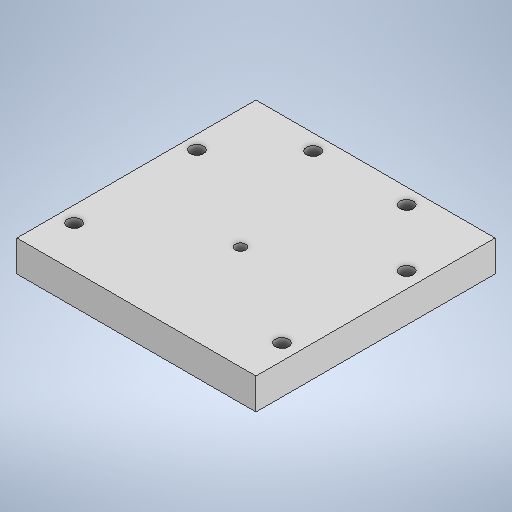
# Autodesk Inventor part: Part_side
Saved by Autodesk Inventor 2025 (Build 290162010, 162A)
## iProperties
Created: 2024-07-05
Part Number: Part_side
Material: Generic
Document SubType Name: Modeling
Designer: kani2
Density: 1 g/cm^3
Appearance: Default
Author: kani2
Autodesk Inventor part; units mm, degrees
ref_plane "YZ Plane" through (0, 0, 0) normal (1, 0, 0) x (0, 1, 0)
ref_plane "XZ Plane" through (0, 0, 0) normal (0, 1, 0) x (-1, 0, 0)
ref_plane "XY Plane" through (0, 0, 0) normal (0, 0, 1) x (1, 0, 0)
sketch "Sketch1" plane through (0, 0, 0) normal (0, 1, 0) x (-1, 0, 0)
  line L0 (73.025, 73.025) -> (-73.025, 73.025)
  line L1 (-73.025, 73.025) -> (-73.025, -73.025)
  line L2 (-73.025, -73.025) -> (73.025, -73.025)
  line L3 (73.025, -73.025) -> (73.025, 73.025)
  line L4 (73.025, 73.025) -> (-73.025, -73.025) construction
  line L5 (-73.025, 73.025) -> (73.025, -73.025) construction
  point P0 (0, 0)
  dimension "d2" = 146.05
  dimension "d3" = 146.05
  constraints: 12 end point, 2 midpoint, 2 parallel, 1 horizontal, 1 perpendicular
  measures "d2" distance of L2.end L1.end
  measures "d3" distance of L1.end L0.end
extrude "Extrusion1" add sketch "Sketch1" along normal blind 19.05
sketch "Sketch2" plane through (0, 19.05, 0) normal (0, 1, 0) x (1, 0, 0)
  circle A0 centre (0, -9.525) radius 3.175
  line L0 (73.025, 73.025) -> (-73.025, 73.025) projected
  line L1 (-73.025, 73.025) -> (-73.025, -73.025) projected
  point P0 (0, 0)
  dimension "d6" = 6.35
  dimension "d7" = 82.55
  dimension "d8" = 73.025
  constraints: 1 centre point
  measures "d6" diameter of A0
  measures "d7" distance from line of L0 A0.centre
  measures "d8" distance from line of L1 A0.centre
extrude "Extrusion2" cut sketch "Sketch2" against normal blind 19.05
sketch "Sketch3" plane through (0, 19.05, 0) normal (0, 1, 0) x (1, 0, 0)
  circle A0 centre (-63.5, -47.625) radius 4.0894
  line L0 (-73.025, 73.025) -> (-73.025, -73.025) projected
  line L1 (-73.025, -73.025) -> (73.025, -73.025) projected
  circle A1 centre (-64.6763, 28.575) radius 4.0894
  circle A2 centre (63.5, -47.625) radius 4.0894
  line L2 (73.025, -73.025) -> (73.025, 73.025) projected
  circle A3 centre (63.5, 28.575) radius 4.0894
  circle A4 centre (-28.575, 63.5) radius 4.0894
  line L3 (73.025, 73.025) -> (-73.025, 73.025) projected
  circle A5 centre (28.575, 63.5) radius 4.0894
  point P0 (0, 0)
  dimension "d11" = 8.1788
  dimension "d12" = 9.525
  dimension "d13" = 25.4
  dimension "d14" = 8.1788
  dimension "d15" = 101.6
  dimension "d16" = 8.1788
  dimension "d17" = 25.4
  dimension "d18" = 9.525
  dimension "d19" = 8.1788
  dimension "d20" = 9.525
  dimension "d21" = 101.6
  dimension "d22" = 8.1788
  dimension "d23" = 44.45
  dimension "d24" = 9.525
  dimension "d25" = 8.1788
  dimension "d26" = 101.6
  constraints: 6 centre point
  measures "d11" diameter of A0
  measures "d12" distance from line of L0 A0.centre
  measures "d13" distance from line of L1 A0.centre
  measures "d14" diameter of A1
  measures "d15" distance from line of L1 A1.centre
  measures "d16" diameter of A2
  measures "d17" distance from line of L1 A2.centre
  measures "d18" distance from line of L2 A2.centre
  measures "d19" diameter of A3
  measures "d20" distance from line of L2 A3.centre
  measures "d21" distance from line of L1 A3.centre
  measures "d22" diameter of A4
  measures "d23" distance from line of L0 A4.centre
  measures "d24" distance from line of L3 A4.centre
  measures "d25" diameter of A5
  measures "d26" distance from line of L0 A5.centre
extrude "Extrusion3" cut sketch "Sketch3" against normal blind 19.05 contours A0 | A1 | A2 | A3 | A4 | A5
body "Solid1"
